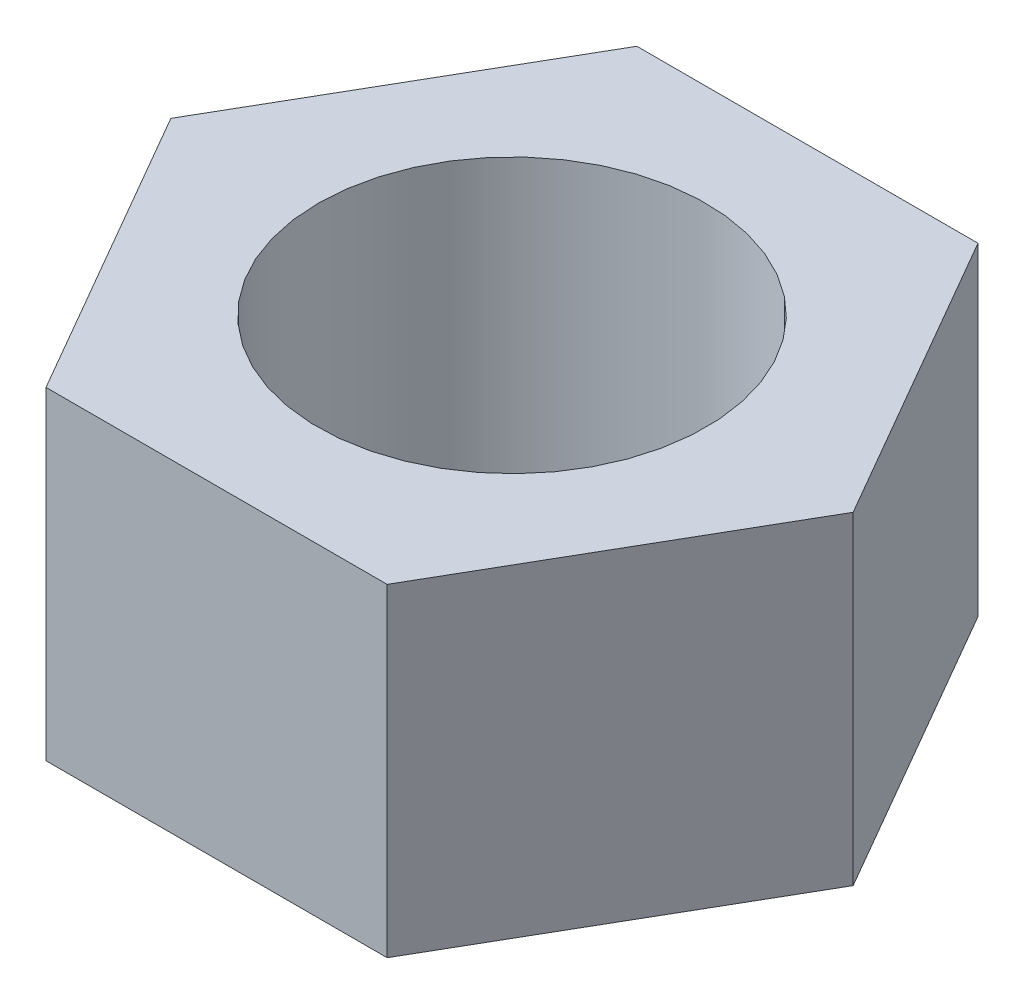
# Autodesk Inventor part: KB33-046-002-003 - Фиксирующая гайка
Saved by Autodesk Inventor 2020 (Build 240168000, 168)
## iProperties
Created: 2021-06-25
Part Number: KB33-046-002-003 - Фиксирующая гайка
Material: Типовые
Document SubType Name: Modeling
Designer: Петров Иван
Mass: 1.76075 g
Surface Area: 13.6214 cm^2
Volume: 1.76075 cm^3
Density: 1 g/cm^3
Appearance: По умолчанию
Author: Петров Иван
Autodesk Inventor part; units mm, degrees
ref_plane "YZ Plane" through (0, 0, 0) normal (1, 0, 0) x (0, 1, 0)
ref_plane "XZ Plane" through (0, 0, 0) normal (0, 1, 0) x (-1, 0, 0)
ref_plane "XY Plane" through (0, 0, 0) normal (0, 0, 1) x (1, 0, 0)
sketch "Эскиз1" plane through (0, 0, 0) normal (0, 1, 0) x (-1, 0, 0)
  line L0 (10.55, 0) -> (5.275, -9.1366)
  line L1 (5.275, -9.1366) -> (-5.275, -9.1366)
  line L2 (-5.275, -9.1366) -> (-10.55, 0)
  line L3 (-10.55, 0) -> (-5.275, 9.1366)
  line L4 (-5.275, 9.1366) -> (5.275, 9.1366)
  line L5 (5.275, 9.1366) -> (10.55, 0)
  circle A0 centre (0, 0) radius 6
  dimension "d0" = 21.1
  dimension "d1" = 12
  constraints: 12 end point, 2 coincident, 1 centre point, 13 other
  measures "d0" distance of L2.end L0.start
  measures "d1" diameter of A0
extrude "Выдавливание1" add sketch "Эскиз1" along normal blind 10
thread "Резьба1" size "M12x1.75" class "6H" standard "ANSI Metric M Profile" full length
